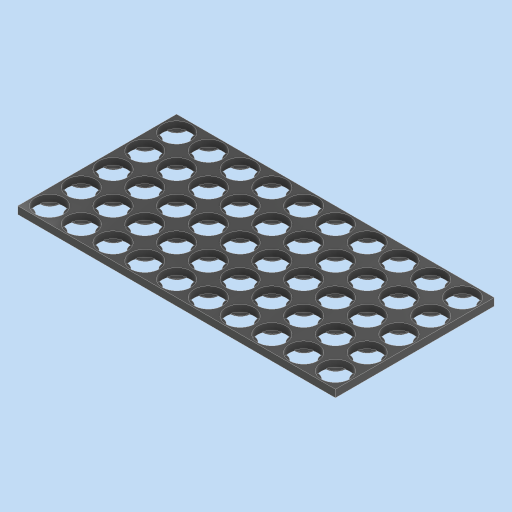
# Autodesk Inventor part: CO-1-1_CellSpacer10by5
Saved by Autodesk Inventor 2023 (Build 270158000, 158)
## iProperties
Created: 2022-10-25
Part Number: CO-1-1_CellSpacer10by5
Material: Generic
Document SubType Name: Modeling
Designer: asach
Density: 1 g/cm^3
Appearance: Dark Gray
Author: asach
Autodesk Inventor part; units mm, degrees
ref_plane "YZ Plane" through (0, 0, 0) normal (1, 0, 0) x (0, 1, 0)
ref_plane "XZ Plane" through (0, 0, 0) normal (0, 1, 0) x (-1, 0, 0)
ref_plane "XY Plane" through (0, 0, 0) normal (0, 0, 1) x (1, 0, 0)
sketch "Sketch1" plane through (0, 0, 0) normal (0, 1, 0) x (-1, 0, 0)
  circle A0 centre (0, 0) radius 10.5
  line L0 (-11.7, 11.7) -> (11.7, 11.7)
  line L1 (11.7, 11.7) -> (11.7, -11.7)
  line L2 (11.7, -11.7) -> (-11.7, -11.7)
  line L3 (-11.7, -11.7) -> (-11.7, 11.7)
  line L4 (-11.7, 11.7) -> (11.7, -11.7) construction
  line L5 (11.7, 11.7) -> (-11.7, -11.7) construction
  line L6 (-10.4975, -0.2304) -> (0.2823, 10.4962)
  line L7 (-11.7, 3.294) -> (-3.0039, 11.7)
  arc A1 (-11.7, 3.294) -> (-3.0039, 11.7) centre (-10.1198, 10.3604) ccw
  arc A2 (-3.294, -11.7) -> (-11.7, -3.0039) centre (-10.3604, -10.1198) ccw
  line L8 (-3.294, -11.7) -> (-11.7, -3.0039)
  arc A3 (11.7, -3.294) -> (3.0039, -11.7) centre (10.1198, -10.3604) ccw
  line L9 (11.7, -3.294) -> (3.0039, -11.7)
  arc A4 (3.294, 11.7) -> (11.7, 3.0039) centre (10.3604, 10.1198) ccw
  line L10 (3.294, 11.7) -> (11.7, 3.0039)
  point P0 (-2.8837, 10.0963)
  point P1 (3.1201, 10.0257)
  point P2 (10.0963, 2.8837)
  point P3 (10.0257, -3.1201)
  point P4 (2.8837, -10.0963)
  point P5 (-3.1201, -10.0257)
  point P6 (-10.0963, -2.8837)
  point P7 (-10.0257, 3.1201)
  dimension "d0" = 21
  dimension "d1" = 23.4
  dimension "d6" = 360
  constraints: 22 end point, 10 point on circle, 5 centre point, 2 midpoint, 2 parallel, 2 perpendicular, 2 point on line, 2 tangent, 1 coincident, 1 horizontal, 21 other
  measures "d0" diameter of A0
  measures "d1" distance of L0.end L1.end
extrude "Extrusion1" add sketch "Sketch1" along normal blind 5 contours A0 A4 L1 A3 | A0 L10 A4 | A3 L9 A0 | A0 A4 L10 | L10 L0 L1 | A0 A1 L0 A4 | L9 A3 A0 | L9 L1 L2 | A3 L2 A2 A0 | A2 L8 A0 | L7 L3 L0 | A1 A0 L7 | L2 L3 L8 | L8 A2 A0 | A2 L3 A1 A0 | A0 A1 L7
extrude "Extrusion2" add sketch "Sketch1" against normal blind 0.5 contours A0 A4 L1 A3 | A4 A0 | A0 L10 A4 | A3 L9 A0 | A0 A3 | A0 A4 L10 | L10 L0 L1 | A0 A1 L0 A4 | L9 A3 A0 | L9 L1 L2 | A3 L2 A2 A0 | A2 L8 A0 | A0 A2 | L7 L3 L0 | A1 A0 L7 | A1 A0 | L2 L3 L8 | L8 A2 A0 | A2 L3 A1 A0 | A0 A1 L7
pattern_linear "Rectangular Pattern1" count 10 spacing 23.4 along (1, 0, 0) count 5 spacing 23.4 along (0, 0, 1)
equation "\"cellSpacing\" = 1.2"
body "Solid1"
